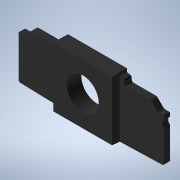
# Autodesk Inventor part: ETH2-17-BC-L_5
Saved by Autodesk Inventor 2021 (Build 250183000, 183)
## iProperties
Created: 2025-05-01
Part Number: ETH2-17-BC-L_5
Material: Generic
Catalog Web Link: www.cadenas.de
Description: ETH2_17_5-ETH2
Vendor: TOYO
Document SubType Name: Modeling
Designer: psAdmin
Manufacturer: TOYO
Mass: 74.9421 g
Surface Area: 210.819 cm^2
Volume: 74.9421 cm^3
Density: 1 g/cm^3
Appearance: PSOLRGB-175-175-175
Category: PARTsolutions
Company: TOYO
Title: ETH2-17-BC-L
Author: Cadenas PARTsolutions
Comments: ETH2
PSOL_IDENT_0: {$CADENAS_DATA/23d-libs/toyo/eth2_series/eth2_17/parts/eth2_17_body5.prj},174 {VTYP=3D},{NB=ETH2-17-
PSOL_IDENT_1: BC-L_5},{LINA=ETH2-17-BC-L},{NN=ETH2_17_5},{DATE=02.07.2024 05:59:00},{GEOMDATE=07.06.2024 03:33:00}
PSOL_IDENT_2: ,{VERSION=},{LINEID=10},{WBVAR=MP,SD},{WBNUMERIC=}  {NB=ETH2-17-BC-L_5},{LINA=ETH2-17-BC-L},{KT=DUMM
PSOL_IDENT_3: Y},{CNSORDERNO=ETH2-17-BC-L},{MODEL=ETH2-17},{MP=BC},{SD=L}
NB: ETH2-17-BC-L_5
NN: ETH2_17_5
NT: ETH2
NBSYN: $CNSORDERNO._5
LINA: ETH2-17-BC-L
CATALOG: TOYO
MODEL: ETH2-17
MP: BC:Motor Exposed
SD: L: Left side of slide
SUPPLIER: TOYO
ARTICLENO: ETH2-17-BC-L_5
BOMINFO: ETH2-17-BC-L
CREATOR: CADENAS GmbH
Autodesk Inventor part; units mm, degrees
sketch "__1" plane through (0, 0, 0) normal (0, 0, 1) x (1, 0, 0)
  line L0 (-75.035, 43.97) -> (-75.035, 2)
  arc A0 (-75.035, 2) -> (-73.035, 0) centre (-73.035, 2) ccw
  line L1 (-73.035, 0) -> (73.035, 0)
  arc A1 (73.035, 0) -> (75.035, 2) centre (73.035, 2) ccw
  line L2 (75.035, 2) -> (75.035, 33.5658)
  arc A2 (75.035, 33.5658) -> (74.7421, 34.2729) centre (74.035, 33.5658) ccw
  line L3 (74.7421, 34.2729) -> (73.8708, 35.1442)
  arc A3 (73.285, 36.5584) -> (73.8708, 35.1442) centre (75.285, 36.5584) ccw
  line L4 (73.285, 36.5584) -> (73.285, 38.4016)
  arc A4 (73.8708, 39.8158) -> (73.285, 38.4016) centre (75.285, 38.4016) ccw
  line L5 (73.8708, 39.8158) -> (74.7421, 40.6871)
  arc A5 (74.7421, 40.6871) -> (75.035, 41.3942) centre (74.035, 41.3942) ccw
  line L6 (75.035, 41.3942) -> (75.035, 43.97)
  arc A6 (75.035, 43.97) -> (74.035, 44.97) centre (74.035, 43.97) ccw
  line L7 (74.035, 44.97) -> (70.2376, 44.97)
  arc A7 (68.1163, 45.8487) -> (70.2376, 44.97) centre (70.2376, 47.97) ccw
  line L8 (68.1163, 45.8487) -> (62.3737, 51.5913)
  arc A8 (62.3737, 51.5913) -> (60.2524, 52.47) centre (60.2524, 49.47) ccw
  line L9 (60.2524, 52.47) -> (37.485, 52.47)
  arc A9 (35.485, 54.47) -> (37.485, 52.47) centre (37.485, 54.47) ccw
  line L10 (35.485, 54.47) -> (35.485, 56.24)
  arc A10 (35.485, 56.24) -> (34.065, 57.96) centre (33.4947, 56.043) ccw
  line L11 (34.065, 57.96) -> (30.735, 58.57)
  line L12 (30.735, 58.57) -> (30.735, 61)
  arc A11 (30.735, 61) -> (29.735, 62) centre (29.735, 61) ccw
  line L13 (29.735, 62) -> (-29.735, 62)
  arc A12 (-29.735, 62) -> (-30.735, 61) centre (-29.735, 61) ccw
  line L14 (-30.735, 61) -> (-30.735, 58.57)
  line L15 (-30.735, 58.57) -> (-34.065, 57.96)
  arc A13 (-34.065, 57.96) -> (-35.485, 56.24) centre (-33.4947, 56.043) ccw
  line L16 (-35.485, 56.24) -> (-35.485, 54.47)
  arc A14 (-37.485, 52.47) -> (-35.485, 54.47) centre (-37.485, 54.47) ccw
  line L17 (-37.485, 52.47) -> (-60.2524, 52.47)
  arc A15 (-60.2524, 52.47) -> (-62.3737, 51.5913) centre (-60.2524, 49.47) ccw
  line L18 (-62.3737, 51.5913) -> (-68.1163, 45.8487)
  arc A16 (-70.2376, 44.97) -> (-68.1163, 45.8487) centre (-70.2376, 47.97) ccw
  line L19 (-70.2376, 44.97) -> (-74.035, 44.97)
  arc A17 (-74.035, 44.97) -> (-75.035, 43.97) centre (-74.035, 43.97) ccw
  circle A18 centre (0, 31.48) radius 16.5
  constraints: 40 end point, 36 point on circle, 19 centre point
extrude "Extrusion1" add sketch "__1" along normal blind 15
sketch "__3" plane through (0, 0, 0) normal (0, 1, 0) x (-1, 0, 0)
  line L0 (80, 6.03) -> (80, 18)
  line L1 (80, 18) -> (-80, 18)
  line L2 (-80, 18) -> (-80, 6.03)
  line L3 (-80, 6.03) -> (-30.735, 7.55)
  line L4 (-30.735, 7.55) -> (-30.28, 15)
  line L5 (-30.28, 15) -> (30.28, 15)
  line L6 (30.28, 15) -> (30.735, 7.55)
  line L7 (30.735, 7.55) -> (80, 6.03)
  constraints: 16 end point
extrude "Extrusion2" cut sketch "__3" along normal blind 61.97
sketch "__4" plane through (0, 0, 0) normal (1, 0, 0) x (0, 1, 0)
  line L0 (63.944, 20) -> (0, 20)
  line L1 (0, 20) -> (0, 0)
  line L2 (0, 0) -> (0.46, 15)
  line L3 (0.46, 15) -> (61.51, 15)
  line L4 (61.51, 15) -> (61.97, 0)
  line L5 (61.97, 0) -> (63.944, 0)
  line L6 (63.944, 0) -> (63.944, 20)
  constraints: 14 end point
extrude "Extrusion3" cut sketch "__4" along normal mid plane 150.07
ref_plane "BODY5_XY" through (0, 0, 0) normal (0, 0, 1) x (1, 0, 0)
ref_plane "BODY5_YZ" through (0, 0, 0) normal (1, 0, 0) x (0, 1, 0)
ref_plane "BODY5_ZX" through (0, 0, 0) normal (0, 1, 0) x (0, 0, 1)
ref_plane "MD1_XY" through (0, 31.48, 15) normal (0, 0, -1) x (1, 0, 0)
ref_plane "MD1_YZ" through (0, 31.48, 15) normal (1, 0, 0) x (0, -1, 0)
ref_plane "MD1_ZX" through (0, 31.48, 15) normal (0, -1, 0) x (0, 0, -1)
body "Solid1"
